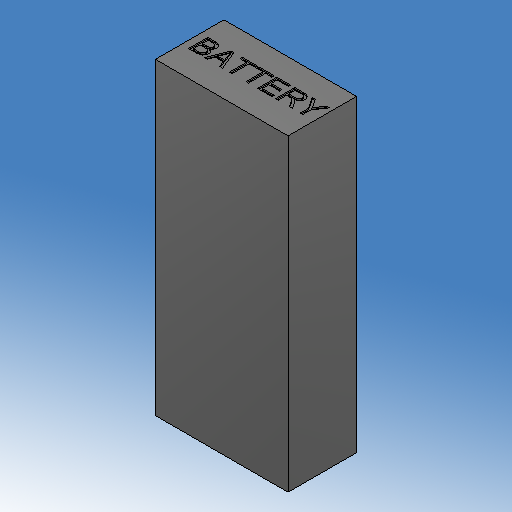
# Autodesk Inventor part: MainBattery
Saved by Autodesk Inventor 2025 (Build 290162000, 162)
## iProperties
Created: 2022-10-07
Part Number: MainBattery
Material: Generic
Document SubType Name: Modeling
Designer: Nebil
Mass: 7634 g
Surface Area: 1557.88 cm^2
Volume: 3445.03 cm^3
Density: 2.21594 g/cm^3
Appearance: Smooth - Black
Author: Nebil
Autodesk Inventor part; units mm, degrees
note: some values were not read from the file. Chosen so that the rebuilt part matches the saved one: direction of "Emboss1".
ref_plane "YZ Plane" through (0, 0, 0) normal (1, 0, 0) x (0, 1, 0)
ref_plane "XZ Plane" through (0, 0, 0) normal (0, 1, 0) x (-1, 0, 0)
ref_plane "XY Plane" through (0, 0, 0) normal (0, 0, 1) x (1, 0, 0)
sketch "Sketch2" plane through (0, 0, 0) normal (0, 1, 0) x (-1, 0, 0)
  line L0 (76.5, -39.5) -> (-76.5, -39.5)
  line L1 (-76.5, -39.5) -> (-76.5, 39.5)
  line L2 (-76.5, 39.5) -> (76.5, 39.5)
  line L3 (76.5, 39.5) -> (76.5, -39.5)
  line L4 (76.5, -39.5) -> (-76.5, 39.5) construction
  line L5 (-76.5, -39.5) -> (76.5, 39.5) construction
  point P0 (0, 0)
  dimension "d0" = 153
  dimension "d1" = 79
  constraints: 12 end point, 2 midpoint, 2 parallel, 1 horizontal, 1 perpendicular
  measures "d0" distance of L1.end L2.end
  measures "d1" distance of L0.end L1.end
extrude "Extrusion1" add sketch "Sketch2" along normal blind 356
sketch "Sketch3" plane through (0, 356, 0) normal (0, 1, 0) x (1, 0, 0)
  line L0 (-71.8667, 17.4104) -> (74.1833, 17.4104) construction
  line L1 (74.1833, 17.4104) -> (74.1833, -14.3396) construction
  line L2 (74.1833, -14.3396) -> (-71.8667, -14.3396) construction
  line L3 (-71.8667, -14.3396) -> (-71.8667, 17.4104) construction
  line L4 (76.5, -39.5) -> (76.5, 39.5) projected
  line L5 (76.5, 39.5) -> (-76.5, 39.5) projected
  line L6 (-76.5, -39.5) -> (76.5, -39.5) projected
  line L7 (-68.1932, -9.5771) -> (-68.1932, 12.6479)
  line L8 (-68.1932, 12.6479) -> (-59.8588, 12.6479)
  spline S0 degree 2 poles (-59.8588, 12.6479) (-57.3178, 12.6479) (-54.2348, 11.2928) (-52.49, 8.4977) (-52.49, 6.9562) knots 0 0 0 1 2 3 3 3
  spline S1 degree 2 poles (-52.49, 6.9562) (-52.49, 5.5332) (-54.0315, 3.0261) (-55.6069, 2.2469) knots 0 0 0 1 2 2 2
  spline S2 degree 2 poles (-55.6069, 2.2469) (-53.5741, 1.654) (-51.4058, -1.1919) (-51.4058, -3.1399) knots 0 0 0 1 2 2 2
  spline S3 degree 2 poles (-51.4058, -3.1399) (-51.4058, -4.6984) (-52.7271, -7.3749) (-54.6583, -8.8317) (-57.5888, -9.5771) (-59.7233, -9.5771) knots 0 0 0 1 2 3 4 4 4
  line L9 (-59.7233, -9.5771) -> (-68.1932, -9.5771)
  line L10 (-65.2456, -6.9514) -> (-59.7063, -6.9514)
  spline S4 degree 2 poles (-59.7063, -6.9514) (-58.2834, -6.9514) (-57.7074, -6.8497) knots 0 0 0 1 1 1
  spline S5 degree 2 poles (-57.7074, -6.8497) (-56.691, -6.6634) (-55.3189, -5.8164) (-54.438, -4.1902) (-54.438, -3.123) knots 0 0 0 1 2 3 3 3
  spline S6 degree 2 poles (-54.438, -3.123) (-54.438, -1.8864) (-55.7424, -0.0569) (-57.9954, 0.6885) (-60.1129, 0.6885) knots 0 0 0 1 2 3 3 3
  line L11 (-60.1129, 0.6885) -> (-65.2456, 0.6885)
  line L12 (-65.2456, 0.6885) -> (-65.2456, -6.9514)
  line L13 (-65.2456, 3.3141) -> (-60.4517, 3.3141)
  spline S7 degree 2 poles (-60.4517, 3.3141) (-58.4867, 3.3141) (-57.6397, 3.5682) knots 0 0 0 1 1 1
  spline S8 degree 2 poles (-57.6397, 3.5682) (-56.5216, 3.907) (-55.3867, 5.4485) (-55.3867, 6.6174) knots 0 0 0 1 2 2 2
  spline S9 degree 2 poles (-55.3867, 6.6174) (-55.3867, 7.7185) (-56.4539, 9.3955) (-58.4189, 10.0223) (-60.8074, 10.0223) knots 0 0 0 1 2 3 3 3
  line L14 (-60.8074, 10.0223) -> (-65.2456, 10.0223)
  line L15 (-65.2456, 10.0223) -> (-65.2456, 3.3141)
  line L16 (-49.7796, -9.5771) -> (-41.242, 12.6479)
  line L17 (-41.242, 12.6479) -> (-38.0573, 12.6479)
  line L18 (-38.0573, 12.6479) -> (-28.9775, -9.5771)
  line L19 (-28.9775, -9.5771) -> (-32.3316, -9.5771)
  line L20 (-32.3316, -9.5771) -> (-34.9065, -2.852)
  line L21 (-34.9065, -2.852) -> (-44.2234, -2.852)
  line L22 (-44.2234, -2.852) -> (-46.6627, -9.5771)
  line L23 (-46.6627, -9.5771) -> (-49.7796, -9.5771)
  line L24 (-43.3764, -0.4634) -> (-35.8212, -0.4634)
  line L25 (-35.8212, -0.4634) -> (-38.1589, 5.7026)
  spline S10 degree 2 poles (-38.1589, 5.7026) (-39.2092, 8.5146) (-39.7174, 10.3103) knots 0 0 0 1 1 1
  spline S11 degree 2 poles (-39.7174, 10.3103) (-40.1578, 8.1758) (-40.9201, 6.0584) knots 0 0 0 1 1 1
  line L26 (-40.9201, 6.0584) -> (-43.3764, -0.4634)
  line L27 (-20.982, -9.5771) -> (-20.982, 10.0223)
  line L28 (-20.982, 10.0223) -> (-28.3, 10.0223)
  line L29 (-28.3, 10.0223) -> (-28.3, 12.6479)
  line L30 (-28.3, 12.6479) -> (-10.6826, 12.6479)
  line L31 (-10.6826, 12.6479) -> (-10.6826, 10.0223)
  line L32 (-10.6826, 10.0223) -> (-18.0344, 10.0223)
  line L33 (-18.0344, 10.0223) -> (-18.0344, -9.5771)
  line L34 (-18.0344, -9.5771) -> (-20.982, -9.5771)
  line L35 (-2.0094, -9.5771) -> (-2.0094, 10.0223)
  line L36 (-2.0094, 10.0223) -> (-9.3274, 10.0223)
  line L37 (-9.3274, 10.0223) -> (-9.3274, 12.6479)
  line L38 (-9.3274, 12.6479) -> (8.29, 12.6479)
  line L39 (8.29, 12.6479) -> (8.29, 10.0223)
  line L40 (8.29, 10.0223) -> (0.9381, 10.0223)
  line L41 (0.9381, 10.0223) -> (0.9381, -9.5771)
  line L42 (0.9381, -9.5771) -> (-2.0094, -9.5771)
  line L43 (11.373, -9.5771) -> (11.373, 12.6479)
  line L44 (11.373, 12.6479) -> (27.4658, 12.6479)
  line L45 (27.4658, 12.6479) -> (27.4658, 10.0223)
  line L46 (27.4658, 10.0223) -> (14.3206, 10.0223)
  line L47 (14.3206, 10.0223) -> (14.3206, 3.2294)
  line L48 (14.3206, 3.2294) -> (26.6358, 3.2294)
  line L49 (26.6358, 3.2294) -> (26.6358, 0.6038)
  line L50 (26.6358, 0.6038) -> (14.3206, 0.6038)
  line L51 (14.3206, 0.6038) -> (14.3206, -6.9514)
  line L52 (14.3206, -6.9514) -> (27.974, -6.9514)
  line L53 (27.974, -6.9514) -> (27.974, -9.5771)
  line L54 (27.974, -9.5771) -> (11.373, -9.5771)
  line L55 (32.0734, -9.5771) -> (32.0734, 12.6479)
  line L56 (32.0734, 12.6479) -> (41.9324, 12.6479)
  spline S12 degree 2 poles (41.9324, 12.6479) (44.8969, 12.6479) (47.9968, 11.4452) (49.8433, 8.413) (49.8433, 6.5835) knots 0 0 0 1 2 3 3 3
  spline S13 degree 2 poles (49.8433, 6.5835) (49.8433, 4.2119) (46.7772, 0.9764) (43.5925, 0.536) knots 0 0 0 1 2 2 2
  spline S14 degree 2 poles (43.5925, 0.536) (44.7444, -0.023) (45.3542, -0.5651) knots 0 0 0 1 1 1
  spline S15 degree 2 poles (45.3542, -0.5651) (46.6417, -1.7509) (47.7936, -3.5295) knots 0 0 0 1 1 1
  line L57 (47.7936, -3.5295) -> (51.6389, -9.5771)
  line L58 (51.6389, -9.5771) -> (47.963, -9.5771)
  line L59 (47.963, -9.5771) -> (45.0154, -4.9525)
  spline S16 degree 2 poles (45.0154, -4.9525) (43.728, -2.9536) (42.0679, -0.8361) (40.7466, 0.0278) (40.069, 0.1972) knots 0 0 0 1 2 3 3 3
  spline S17 degree 2 poles (40.069, 0.1972) (39.5608, 0.2988) (38.4259, 0.2988) knots 0 0 0 1 1 1
  line L60 (38.4259, 0.2988) -> (35.021, 0.2988)
  line L61 (35.021, 0.2988) -> (35.021, -9.5771)
  line L62 (35.021, -9.5771) -> (32.0734, -9.5771)
  line L63 (35.021, 2.8398) -> (41.3395, 2.8398)
  spline S18 degree 2 poles (41.3395, 2.8398) (43.3553, 2.8398) (45.6253, 3.6699) (46.8111, 5.5163) (46.8111, 6.5835) knots 0 0 0 1 2 3 3 3
  spline S19 degree 2 poles (46.8111, 6.5835) (46.8111, 8.1589) (44.5242, 10.1917) (42.051, 10.1917) knots 0 0 0 1 2 2 2
  line L64 (42.051, 10.1917) -> (35.021, 10.1917)
  line L65 (35.021, 10.1917) -> (35.021, 2.8398)
  line L66 (60.7186, -9.5771) -> (60.7186, -0.1585)
  line L67 (60.7186, -0.1585) -> (52.1471, 12.6479)
  line L68 (52.1471, 12.6479) -> (55.7214, 12.6479)
  line L69 (55.7214, 12.6479) -> (60.1088, 5.9398)
  spline S20 degree 2 poles (60.1088, 5.9398) (61.3454, 4.0764) (62.3787, 2.1792) knots 0 0 0 1 1 1
  spline S21 degree 2 poles (62.3787, 2.1792) (63.3782, 3.924) (64.8011, 6.1092) knots 0 0 0 1 1 1
  line L70 (64.8011, 6.1092) -> (69.1208, 12.6479)
  line L71 (69.1208, 12.6479) -> (72.5426, 12.6479)
  line L72 (72.5426, 12.6479) -> (63.6662, -0.1585)
  line L73 (63.6662, -0.1585) -> (63.6662, -9.5771)
  line L74 (63.6662, -9.5771) -> (60.7186, -9.5771)
  point P0 (0, 0)
  dimension "d4" = 146.05
  dimension "d5" = 2.3167
  dimension "d6" = 22.0895
  dimension "d8" = 31.75
  constraints: 2 other
  measures "d4" distance of L1.end L2.end
  measures "d5" distance between parallel lines of L4 L1
  measures "d6" distance between parallel lines of L5 L0
  measures "d8" distance of L2.end L0.start
emboss "Emboss1" sketch "Sketch3" operation cut depth 1.5875 direction (0, -1, 0)
equation "\"d5\" = -0.333333 * d4 + 0.333333 * d0"
equation "\"d6\" = -0.298507 * d1 + 0.298507 * d0"
body "Solid1"
